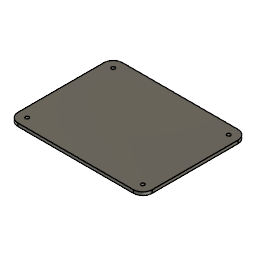
bottom_plate_macropad (Autodesk Fusion 360 design; units mm, degrees)
part number: 2026-03-29-12-35-56-853
Autodesk Fusion 360 part; units mm, degrees
sketch "Sketch1" plane through (0, 0, 0) normal (0, 0, 1) x (1, 0, 0)
  line L0 (0, 0) -> (86.2, 0)
  line L1 (86.2, 0) -> (86.2, -67.2)
  line L2 (86.2, -67.2) -> (0, -67.2)
  line L3 (0, -67.2) -> (0, 0)
  dimension "d1" = 86.2
  dimension "d2" = 67.2
  constraint horizontal L0
  constraint vertical L1
  constraint horizontal L2
  constraint vertical L3
  constraint coincident L0.start L3.end
  measures "d1" distance of L0.start L0.end
  measures "d2" distance of L0.start L2.end
extrude "Extrude1" add sketch "Sketch1" along normal blind 2
fillet "Fillet1" radius 6 4 edges at (0, 0, 1) (0, -67.2, 1) (86.2, -67.2, 1) (86.2, 0, 1)
sketch "Sketch2" plane through (0, 0, 2) normal (0, 0, 1) x (-1, 0, 0)
  arc A0 (-86.2, 6) -> (-80.2, 0) centre (-80.2, 6) ccw
  line L0 (-80.2, 0) -> (-6, 0)
  arc A1 (-6, 0) -> (0, 6) centre (-6, 6) ccw
  line L1 (0, 6) -> (0, 61.2)
  arc A2 (0, 61.2) -> (-6, 67.2) centre (-6, 61.2) ccw
  line L2 (-6, 67.2) -> (-80.2, 67.2)
  arc A3 (-80.2, 67.2) -> (-86.2, 61.2) centre (-80.2, 61.2) ccw
  line L3 (-86.2, 61.2) -> (-86.2, 6)
  circle A4 centre (-80.2, 61.2) radius 1.1
  circle A5 centre (-6, 61.2) radius 1.1
  circle A6 centre (-6, 6) radius 1.1
  circle A7 centre (-80.2, 6) radius 1.1
  dimension "d7" = 2.2
  dimension "d8" = 2.2
  dimension "d9" = 2.2
  dimension "d10" = 2.2
  dimension "d11" = 6
  dimension "d12" = 6
  dimension "d13" = 6
  dimension "d14" = 6
  dimension "d15" = 6
  dimension "d16" = 6
  dimension "d17" = 6
  dimension "d18" = 6
  measures "d7" diameter of A4
  measures "d8" diameter of A5
  measures "d9" diameter of A6
  measures "d10" diameter of A7
  measures "d11" distance of L2 A3.centre
  measures "d12" distance of L3 A3.centre
  measures "d13" distance of L1 A2.centre
  measures "d14" distance of L2 A2.centre
  measures "d15" distance of L1 A1.centre
  measures "d16" distance of L0 A1.centre
  measures "d17" distance of L0 A0.centre
  measures "d18" distance of L3 A0.centre
hole "Hole1" at (80.2, -61.2, 2) at (6, -61.2, 2) at (6, -6, 2) at (80.2, -6, 2) direction (0, 0, -1) diameter 2.2 depth 2.2 tip angle 118
